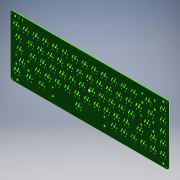
# Autodesk Inventor part: 60pc_pcb.kicad_pcb_Outline
Saved by Autodesk Inventor 2018 (Build 220112000, 112)
## iProperties
Created: 2018-02-05
Part Number: 60pc_pcb.kicad_pcb_Outline
Material: Generic
Document SubType Name: Modeling
Designer: ConnorDevitt
Density: 1 g/cm^3
Appearance: Board Outline
Author: ConnorDevitt
Autodesk Inventor part; units mm, degrees
(part 1 of 2)
ref_plane "YZ Plane" through (0, 0, 0) normal (1, 0, 0) x (0, 1, 0)
ref_plane "XZ Plane" through (0, 0, 0) normal (0, 1, 0) x (-1, 0, 0)
ref_plane "XY Plane" through (0, 0, 0) normal (0, 0, 1) x (1, 0, 0)
sketch "Sketch1" plane through (0, 0, 0) normal (0, 0, 1) x (1, 0, 0)
  line L0 (-153.25, 55.25) -> (-153.25, -54)
  arc A0 (-153.25, -54) -> (-149.25, -58) centre (-149.25, -54) ccw
  line L1 (-149.25, -58) -> (149.25, -58)
  arc A1 (149.25, -58) -> (153.25, -54) centre (149.25, -54) ccw
  line L2 (153.25, -54) -> (153.25, -53.25)
  line L3 (153.25, -53.25) -> (153.25, 55.25)
  arc A2 (153.25, 55.25) -> (150.5, 58) centre (150.5, 55.25) ccw
  line L4 (150.5, 58) -> (-150.5, 58)
  arc A3 (-150.5, 58) -> (-153.25, 55.25) centre (-150.5, 55.25) ccw
  line L5 (-126.1877, 42.5233) -> (-126.9986, 41.0634)
  arc A4 (-128.3099, 41.7917) -> (-126.9986, 41.0634) centre (-127.6542, 41.4275) ccw
  line L6 (-128.3099, 41.7917) -> (-127.4989, 43.2516)
  arc A5 (-126.1877, 42.5233) -> (-127.4989, 43.2516) centre (-126.8433, 42.8875) ccw
  line L7 (-120.5558, 43.9158) -> (-120.5952, 43.3372)
  arc A6 (-122.0917, 43.4392) -> (-120.5952, 43.3372) centre (-121.3435, 43.3882) ccw
  line L8 (-122.0917, 43.4392) -> (-122.0523, 44.0178)
  arc A7 (-120.5558, 43.9158) -> (-122.0523, 44.0178) centre (-121.304, 43.9668) ccw
  line L9 (-136.55, 55.15) -> (-136.55, 52.65)
  arc A8 (-137.25, 52.65) -> (-136.55, 52.65) centre (-136.9, 52.65) ccw
  line L10 (-137.25, 52.65) -> (-137.25, 55.15)
  arc A9 (-136.55, 55.15) -> (-137.25, 55.15) centre (-136.9, 55.15) ccw
  line L11 (-129.25, 55.15) -> (-129.25, 52.65)
  arc A10 (-129.95, 52.65) -> (-129.25, 52.65) centre (-129.6, 52.65) ccw
  line L12 (-129.95, 52.65) -> (-129.95, 55.15)
  arc A11 (-129.25, 55.15) -> (-129.95, 55.15) centre (-129.6, 55.15) ccw
  line L13 (-145.2377, 42.5233) -> (-146.0486, 41.0634)
  arc A12 (-147.3598, 41.7917) -> (-146.0486, 41.0634) centre (-146.7042, 41.4275) ccw
  line L14 (-147.3598, 41.7917) -> (-146.5489, 43.2516)
  arc A13 (-145.2377, 42.5233) -> (-146.5489, 43.2516) centre (-145.8933, 42.8875) ccw
  line L15 (-139.6058, 43.9158) -> (-139.6452, 43.3372)
  arc A14 (-141.1417, 43.4392) -> (-139.6452, 43.3372) centre (-140.3935, 43.3882) ccw
  line L16 (-141.1417, 43.4392) -> (-141.1023, 44.0178)
  arc A15 (-139.6058, 43.9158) -> (-141.1023, 44.0178) centre (-140.354, 43.9668) ccw
  line L17 (-140.4752, 23.4733) -> (-141.2861, 22.0134)
  arc A16 (-142.5974, 22.7417) -> (-141.2861, 22.0134) centre (-141.9417, 22.3775) ccw
  line L18 (-142.5974, 22.7417) -> (-141.7864, 24.2016)
  arc A17 (-140.4752, 23.4733) -> (-141.7864, 24.2016) centre (-141.1308, 23.8375) ccw
  line L19 (-134.8433, 24.8658) -> (-134.8827, 24.2872)
  arc A18 (-136.3792, 24.3892) -> (-134.8827, 24.2872) centre (-135.631, 24.3382) ccw
  line L20 (-136.3792, 24.3892) -> (-136.3398, 24.9678)
  arc A19 (-134.8433, 24.8658) -> (-136.3398, 24.9678) centre (-135.5915, 24.9168) ccw
  line L21 (-138.0939, 4.4233) -> (-138.9048, 2.9634)
  arc A20 (-140.2161, 3.6917) -> (-138.9048, 2.9634) centre (-139.5605, 3.3275) ccw
  line L22 (-140.2161, 3.6917) -> (-139.4052, 5.1516)
  arc A21 (-138.0939, 4.4233) -> (-139.4052, 5.1516) centre (-138.7495, 4.7875) ccw
  line L23 (-132.462, 5.8158) -> (-132.5015, 5.2372)
  arc A22 (-133.998, 5.3392) -> (-132.5015, 5.2372) centre (-133.2497, 5.2882) ccw
  line L24 (-133.998, 5.3392) -> (-133.9585, 5.9178)
  arc A23 (-132.462, 5.8158) -> (-133.9585, 5.9178) centre (-133.2103, 5.8668) ccw
  line L25 (-133.3314, -14.6267) -> (-134.1423, -16.0866)
  arc A24 (-135.4536, -15.3583) -> (-134.1423, -16.0866) centre (-134.798, -15.7225) ccw
  line L26 (-135.4536, -15.3583) -> (-134.6427, -13.8984)
  arc A25 (-133.3314, -14.6267) -> (-134.6427, -13.8984) centre (-133.987, -14.2625) ccw
  line L27 (-127.6995, -13.2342) -> (-127.739, -13.8128)
  arc A26 (-129.2355, -13.7108) -> (-127.739, -13.8128) centre (-128.4872, -13.7618) ccw
  line L28 (-129.2355, -13.7108) -> (-129.196, -13.1322)
  arc A27 (-127.6995, -13.2342) -> (-129.196, -13.1322) centre (-128.4478, -13.1832) ccw
  line L29 (-142.8564, -33.6767) -> (-143.6673, -35.1366)
  arc A28 (-144.9786, -34.4083) -> (-143.6673, -35.1366) centre (-144.323, -34.7725) ccw
  line L30 (-144.9786, -34.4083) -> (-144.1677, -32.9484)
  arc A29 (-142.8564, -33.6767) -> (-144.1677, -32.9484) centre (-143.512, -33.3125) ccw
  line L31 (-137.2245, -32.2842) -> (-137.264, -32.8628)
  arc A30 (-138.7605, -32.7608) -> (-137.264, -32.8628) centre (-138.0122, -32.8118) ccw
  line L32 (-138.7605, -32.7608) -> (-138.721, -32.1822)
  arc A31 (-137.2245, -32.2842) -> (-138.721, -32.1822) centre (-137.9728, -32.2332) ccw
  line L33 (-116.6627, 23.4733) -> (-117.4736, 22.0134)
  arc A32 (-118.7849, 22.7417) -> (-117.4736, 22.0134) centre (-118.1292, 22.3775) ccw
  line L34 (-118.7849, 22.7417) -> (-117.9739, 24.2016)
  arc A33 (-116.6627, 23.4733) -> (-117.9739, 24.2016) centre (-117.3183, 23.8375) ccw
  line L35 (-111.0308, 24.8658) -> (-111.0702, 24.2872)
  arc A34 (-112.5667, 24.3892) -> (-111.0702, 24.2872) centre (-111.8185, 24.3382) ccw
  line L36 (-112.5667, 24.3892) -> (-112.5273, 24.9678)
  arc A35 (-111.0308, 24.8658) -> (-112.5273, 24.9678) centre (-111.779, 24.9168) ccw
  line L37 (-111.9002, 4.4233) -> (-112.7111, 2.9634)
  arc A36 (-114.0224, 3.6917) -> (-112.7111, 2.9634) centre (-113.3667, 3.3275) ccw
  line L38 (-114.0224, 3.6917) -> (-113.2114, 5.1516)
  arc A37 (-111.9002, 4.4233) -> (-113.2114, 5.1516) centre (-112.5558, 4.7875) ccw
  line L39 (-106.2683, 5.8158) -> (-106.3077, 5.2372)
  arc A38 (-107.8042, 5.3392) -> (-106.3077, 5.2372) centre (-107.056, 5.2882) ccw
  line L40 (-107.8042, 5.3392) -> (-107.7648, 5.9178)
  arc A39 (-106.2683, 5.8158) -> (-107.7648, 5.9178) centre (-107.0165, 5.8668) ccw
  line L41 (-102.3752, -14.6267) -> (-103.1861, -16.0866)
  arc A40 (-104.4974, -15.3583) -> (-103.1861, -16.0866) centre (-103.8417, -15.7225) ccw
  line L42 (-104.4974, -15.3583) -> (-103.6864, -13.8984)
  arc A41 (-102.3752, -14.6267) -> (-103.6864, -13.8984) centre (-103.0308, -14.2625) ccw
  line L43 (-96.7433, -13.2342) -> (-96.7827, -13.8128)
  arc A42 (-98.2792, -13.7108) -> (-96.7827, -13.8128) centre (-97.531, -13.7618) ccw
  line L44 (-98.2792, -13.7108) -> (-98.2398, -13.1322)
  arc A43 (-96.7433, -13.2342) -> (-98.2398, -13.1322) centre (-97.4915, -13.1832) ccw
  line L45 (-119.0439, -33.6767) -> (-119.8548, -35.1366)
  arc A44 (-121.1661, -34.4083) -> (-119.8548, -35.1366) centre (-120.5105, -34.7725) ccw
  line L46 (-121.1661, -34.4083) -> (-120.3552, -32.9484)
  arc A45 (-119.0439, -33.6767) -> (-120.3552, -32.9484) centre (-119.6995, -33.3125) ccw
  line L47 (-113.412, -32.2842) -> (-113.4515, -32.8628)
  arc A46 (-114.948, -32.7608) -> (-113.4515, -32.8628) centre (-114.1997, -32.8118) ccw
  line L48 (-114.948, -32.7608) -> (-114.9085, -32.1822)
  arc A47 (-113.412, -32.2842) -> (-114.9085, -32.1822) centre (-114.1603, -32.2332) ccw
  line L49 (-95.2314, -33.6767) -> (-96.0423, -35.1366)
  arc A48 (-97.3536, -34.4083) -> (-96.0423, -35.1366) centre (-96.698, -34.7725) ccw
  line L50 (-97.3536, -34.4083) -> (-96.5427, -32.9484)
  arc A49 (-95.2314, -33.6767) -> (-96.5427, -32.9484) centre (-95.887, -33.3125) ccw
  line L51 (-89.5995, -32.2842) -> (-89.639, -32.8628)
  arc A50 (-91.1355, -32.7608) -> (-89.639, -32.8628) centre (-90.3872, -32.8118) ccw
  line L52 (-91.1355, -32.7608) -> (-91.096, -32.1822)
  arc A51 (-89.5995, -32.2842) -> (-91.096, -32.1822) centre (-90.3478, -32.2332) ccw
  line L53 (-107.1377, 42.5233) -> (-107.9486, 41.0634)
  arc A52 (-109.2599, 41.7917) -> (-107.9486, 41.0634) centre (-108.6042, 41.4275) ccw
  line L54 (-109.2599, 41.7917) -> (-108.4489, 43.2516)
  arc A53 (-107.1377, 42.5233) -> (-108.4489, 43.2516) centre (-107.7933, 42.8875) ccw
  line L55 (-101.5058, 43.9158) -> (-101.5452, 43.3372)
  arc A54 (-103.0417, 43.4392) -> (-101.5452, 43.3372) centre (-102.2935, 43.3882) ccw
  line L56 (-103.0417, 43.4392) -> (-103.0023, 44.0178)
  arc A55 (-101.5058, 43.9158) -> (-103.0023, 44.0178) centre (-102.254, 43.9668) ccw
  line L57 (-97.6127, 23.4733) -> (-98.4236, 22.0134)
  arc A56 (-99.7348, 22.7417) -> (-98.4236, 22.0134) centre (-99.0792, 22.3775) ccw
  line L58 (-99.7348, 22.7417) -> (-98.9239, 24.2016)
  arc A57 (-97.6127, 23.4733) -> (-98.9239, 24.2016) centre (-98.2683, 23.8375) ccw
  line L59 (-91.9808, 24.8658) -> (-92.0202, 24.2872)
  arc A58 (-93.5167, 24.3892) -> (-92.0202, 24.2872) centre (-92.7685, 24.3382) ccw
  line L60 (-93.5167, 24.3892) -> (-93.4773, 24.9678)
  arc A59 (-91.9808, 24.8658) -> (-93.4773, 24.9678) centre (-92.729, 24.9168) ccw
  line L61 (-92.8501, 4.4233) -> (-93.6611, 2.9634)
  arc A60 (-94.9724, 3.6917) -> (-93.6611, 2.9634) centre (-94.3167, 3.3275) ccw
  line L62 (-94.9724, 3.6917) -> (-94.1614, 5.1516)
  arc A61 (-92.8501, 4.4233) -> (-94.1614, 5.1516) centre (-93.5058, 4.7875) ccw
  line L63 (-87.2183, 5.8158) -> (-87.2577, 5.2372)
  arc A62 (-88.7542, 5.3392) -> (-87.2577, 5.2372) centre (-88.006, 5.2882) ccw
  line L64 (-88.7542, 5.3392) -> (-88.7148, 5.9178)
  arc A63 (-87.2183, 5.8158) -> (-88.7148, 5.9178) centre (-87.9665, 5.8668) ccw
  line L65 (-83.3251, -14.6267) -> (-84.1361, -16.0866)
  arc A64 (-85.4474, -15.3583) -> (-84.1361, -16.0866) centre (-84.7917, -15.7225) ccw
  line L66 (-85.4474, -15.3583) -> (-84.6364, -13.8984)
  arc A65 (-83.3251, -14.6267) -> (-84.6364, -13.8984) centre (-83.9808, -14.2625) ccw
  line L67 (-77.6933, -13.2342) -> (-77.7327, -13.8128)
  arc A66 (-79.2292, -13.7108) -> (-77.7327, -13.8128) centre (-78.481, -13.7618) ccw
  line L68 (-79.2292, -13.7108) -> (-79.1898, -13.1322)
  arc A67 (-77.6933, -13.2342) -> (-79.1898, -13.1322) centre (-78.4415, -13.1832) ccw
  line L69 (-88.0876, 42.5233) -> (-88.8986, 41.0634)
  arc A68 (-90.2099, 41.7917) -> (-88.8986, 41.0634) centre (-89.5542, 41.4275) ccw
  line L70 (-90.2099, 41.7917) -> (-89.3989, 43.2516)
  arc A69 (-88.0876, 42.5233) -> (-89.3989, 43.2516) centre (-88.7433, 42.8875) ccw
  line L71 (-82.4558, 43.9158) -> (-82.4952, 43.3372)
  arc A70 (-83.9917, 43.4392) -> (-82.4952, 43.3372) centre (-83.2435, 43.3882) ccw
  line L72 (-83.9917, 43.4392) -> (-83.9523, 44.0178)
  arc A71 (-82.4558, 43.9158) -> (-83.9523, 44.0178) centre (-83.204, 43.9668) ccw
  line L73 (-78.5627, 23.4733) -> (-79.3736, 22.0134)
  arc A72 (-80.6849, 22.7417) -> (-79.3736, 22.0134) centre (-80.0292, 22.3775) ccw
  line L74 (-80.6849, 22.7417) -> (-79.8739, 24.2016)
  arc A73 (-78.5627, 23.4733) -> (-79.8739, 24.2016) centre (-79.2183, 23.8375) ccw
  line L75 (-72.9308, 24.8658) -> (-72.9702, 24.2872)
  arc A74 (-74.4667, 24.3892) -> (-72.9702, 24.2872) centre (-73.7185, 24.3382) ccw
  line L76 (-74.4667, 24.3892) -> (-74.4273, 24.9678)
  arc A75 (-72.9308, 24.8658) -> (-74.4273, 24.9678) centre (-73.679, 24.9168) ccw
  line L77 (-73.8002, 4.4233) -> (-74.6111, 2.9634)
  arc A76 (-75.9223, 3.6917) -> (-74.6111, 2.9634) centre (-75.2667, 3.3275) ccw
  line L78 (-75.9223, 3.6917) -> (-75.1114, 5.1516)
  arc A77 (-73.8002, 4.4233) -> (-75.1114, 5.1516) centre (-74.4558, 4.7875) ccw
  line L79 (-68.1683, 5.8158) -> (-68.2077, 5.2372)
  arc A78 (-69.7042, 5.3392) -> (-68.2077, 5.2372) centre (-68.956, 5.2882) ccw
  line L80 (-69.7042, 5.3392) -> (-69.6648, 5.9178)
  arc A79 (-68.1683, 5.8158) -> (-69.6648, 5.9178) centre (-68.9165, 5.8668) ccw
  line L81 (-64.2751, -14.6267) -> (-65.0861, -16.0866)
  arc A80 (-66.3974, -15.3583) -> (-65.0861, -16.0866) centre (-65.7417, -15.7225) ccw
  line L82 (-66.3974, -15.3583) -> (-65.5864, -13.8984)
  arc A81 (-64.2751, -14.6267) -> (-65.5864, -13.8984) centre (-64.9308, -14.2625) ccw
  line L83 (-58.6433, -13.2342) -> (-58.6827, -13.8128)
  arc A82 (-60.1792, -13.7108) -> (-58.6827, -13.8128) centre (-59.431, -13.7618) ccw
  line L84 (-60.1792, -13.7108) -> (-60.1398, -13.1322)
  arc A83 (-58.6433, -13.2342) -> (-60.1398, -13.1322) centre (-59.3915, -13.1832) ccw
  line L85 (-69.0376, 42.5233) -> (-69.8486, 41.0634)
  arc A84 (-71.1599, 41.7917) -> (-69.8486, 41.0634) centre (-70.5042, 41.4275) ccw
  line L86 (-71.1599, 41.7917) -> (-70.3489, 43.2516)
  arc A85 (-69.0376, 42.5233) -> (-70.3489, 43.2516) centre (-69.6933, 42.8875) ccw
  line L87 (-63.4058, 43.9158) -> (-63.4452, 43.3372)
  arc A86 (-64.9417, 43.4392) -> (-63.4452, 43.3372) centre (-64.1935, 43.3882) ccw
  line L88 (-64.9417, 43.4392) -> (-64.9023, 44.0178)
  arc A87 (-63.4058, 43.9158) -> (-64.9023, 44.0178) centre (-64.154, 43.9668) ccw
  line L89 (-59.5127, 23.4733) -> (-60.3236, 22.0134)
  arc A88 (-61.6349, 22.7417) -> (-60.3236, 22.0134) centre (-60.9792, 22.3775) ccw
  line L90 (-61.6349, 22.7417) -> (-60.8239, 24.2016)
  arc A89 (-59.5127, 23.4733) -> (-60.8239, 24.2016) centre (-60.1683, 23.8375) ccw
  line L91 (-53.8808, 24.8658) -> (-53.9202, 24.2872)
  arc A90 (-55.4167, 24.3892) -> (-53.9202, 24.2872) centre (-54.6685, 24.3382) ccw
  line L92 (-55.4167, 24.3892) -> (-55.3773, 24.9678)
  arc A91 (-53.8808, 24.8658) -> (-55.3773, 24.9678) centre (-54.629, 24.9168) ccw
  line L93 (-54.7501, 4.4233) -> (-55.5611, 2.9634)
  arc A92 (-56.8724, 3.6917) -> (-55.5611, 2.9634) centre (-56.2167, 3.3275) ccw
  line L94 (-56.8724, 3.6917) -> (-56.0614, 5.1516)
  arc A93 (-54.7501, 4.4233) -> (-56.0614, 5.1516) centre (-55.4058, 4.7875) ccw
  line L95 (-49.1183, 5.8158) -> (-49.1577, 5.2372)
  arc A94 (-50.6542, 5.3392) -> (-49.1577, 5.2372) centre (-49.906, 5.2882) ccw
  line L96 (-50.6542, 5.3392) -> (-50.6148, 5.9178)
  arc A95 (-49.1183, 5.8158) -> (-50.6148, 5.9178) centre (-49.8665, 5.8668) ccw
  line L97 (-45.2251, -14.6267) -> (-46.0361, -16.0866)
  arc A96 (-47.3473, -15.3583) -> (-46.0361, -16.0866) centre (-46.6917, -15.7225) ccw
  line L98 (-47.3473, -15.3583) -> (-46.5364, -13.8984)
  arc A97 (-45.2251, -14.6267) -> (-46.5364, -13.8984) centre (-45.8808, -14.2625) ccw
  line L99 (-39.5933, -13.2342) -> (-39.6327, -13.8128)
  arc A98 (-41.1292, -13.7108) -> (-39.6327, -13.8128) centre (-40.381, -13.7618) ccw
  line L100 (-41.1292, -13.7108) -> (-41.0898, -13.1322)
  arc A99 (-39.5933, -13.2342) -> (-41.0898, -13.1322) centre (-40.3415, -13.1832) ccw
  line L101 (-49.9877, 42.5233) -> (-50.7986, 41.0634)
  arc A100 (-52.1099, 41.7917) -> (-50.7986, 41.0634) centre (-51.4542, 41.4275) ccw
  line L102 (-52.1099, 41.7917) -> (-51.2989, 43.2516)
  arc A101 (-49.9877, 42.5233) -> (-51.2989, 43.2516) centre (-50.6433, 42.8875) ccw
  line L103 (-44.3558, 43.9158) -> (-44.3952, 43.3372)
  arc A102 (-45.8917, 43.4392) -> (-44.3952, 43.3372) centre (-45.1435, 43.3882) ccw
  line L104 (-45.8917, 43.4392) -> (-45.8523, 44.0178)
  arc A103 (-44.3558, 43.9158) -> (-45.8523, 44.0178) centre (-45.104, 43.9668) ccw
  line L105 (-40.4626, 23.4733) -> (-41.2736, 22.0134)
  arc A104 (-42.5849, 22.7417) -> (-41.2736, 22.0134) centre (-41.9292, 22.3775) ccw
  line L106 (-42.5849, 22.7417) -> (-41.7739, 24.2016)
  arc A105 (-40.4626, 23.4733) -> (-41.7739, 24.2016) centre (-41.1183, 23.8375) ccw
  line L107 (-34.8308, 24.8658) -> (-34.8702, 24.2872)
  arc A106 (-36.3667, 24.3892) -> (-34.8702, 24.2872) centre (-35.6185, 24.3382) ccw
  line L108 (-36.3667, 24.3892) -> (-36.3273, 24.9678)
  arc A107 (-34.8308, 24.8658) -> (-36.3273, 24.9678) centre (-35.579, 24.9168) ccw
  line L109 (-35.7002, 4.4233) -> (-36.5111, 2.9634)
  arc A108 (-37.8224, 3.6917) -> (-36.5111, 2.9634) centre (-37.1667, 3.3275) ccw
  line L110 (-37.8224, 3.6917) -> (-37.0114, 5.1516)
  arc A109 (-35.7002, 4.4233) -> (-37.0114, 5.1516) centre (-36.3558, 4.7875) ccw
  line L111 (-30.0683, 5.8158) -> (-30.1077, 5.2372)
  arc A110 (-31.6042, 5.3392) -> (-30.1077, 5.2372) centre (-30.856, 5.2882) ccw
  line L112 (-31.6042, 5.3392) -> (-31.5648, 5.9178)
  arc A111 (-30.0683, 5.8158) -> (-31.5648, 5.9178) centre (-30.8165, 5.8668) ccw
  line L113 (-26.1752, -14.6267) -> (-26.9861, -16.0866)
  arc A112 (-28.2974, -15.3583) -> (-26.9861, -16.0866) centre (-27.6417, -15.7225) ccw
  line L114 (-28.2974, -15.3583) -> (-27.4864, -13.8984)
  arc A113 (-26.1752, -14.6267) -> (-27.4864, -13.8984) centre (-26.8308, -14.2625) ccw
  line L115 (-20.5433, -13.2342) -> (-20.5827, -13.8128)
  arc A114 (-22.0792, -13.7108) -> (-20.5827, -13.8128) centre (-21.331, -13.7618) ccw
  line L116 (-22.0792, -13.7108) -> (-22.0398, -13.1322)
  arc A115 (-20.5433, -13.2342) -> (-22.0398, -13.1322) centre (-21.2915, -13.1832) ccw
  line L117 (-30.9377, 42.5233) -> (-31.7486, 41.0634)
  arc A116 (-33.0598, 41.7917) -> (-31.7486, 41.0634) centre (-32.4042, 41.4275) ccw
  line L118 (-33.0598, 41.7917) -> (-32.2489, 43.2516)
  arc A117 (-30.9377, 42.5233) -> (-32.2489, 43.2516) centre (-31.5933, 42.8875) ccw
  line L119 (-25.3058, 43.9158) -> (-25.3452, 43.3372)
  arc A118 (-26.8417, 43.4392) -> (-25.3452, 43.3372) centre (-26.0935, 43.3882) ccw
  line L120 (-26.8417, 43.4392) -> (-26.8023, 44.0178)
  arc A119 (-25.3058, 43.9158) -> (-26.8023, 44.0178) centre (-26.054, 43.9668) ccw
  line L121 (-21.4127, 23.4733) -> (-22.2236, 22.0134)
  arc A120 (-23.5348, 22.7417) -> (-22.2236, 22.0134) centre (-22.8792, 22.3775) ccw
  line L122 (-23.5348, 22.7417) -> (-22.7239, 24.2016)
  arc A121 (-21.4127, 23.4733) -> (-22.7239, 24.2016) centre (-22.0683, 23.8375) ccw
  line L123 (-15.7808, 24.8658) -> (-15.8202, 24.2872)
  arc A122 (-17.3167, 24.3892) -> (-15.8202, 24.2872) centre (-16.5685, 24.3382) ccw
  line L124 (-17.3167, 24.3892) -> (-17.2773, 24.9678)
  arc A123 (-15.7808, 24.8658) -> (-17.2773, 24.9678) centre (-16.529, 24.9168) ccw
  line L125 (-16.6502, 4.4233) -> (-17.4611, 2.9634)
  arc A124 (-18.7723, 3.6917) -> (-17.4611, 2.9634) centre (-18.1167, 3.3275) ccw
  line L126 (-18.7723, 3.6917) -> (-17.9614, 5.1516)
  arc A125 (-16.6502, 4.4233) -> (-17.9614, 5.1516) centre (-17.3058, 4.7875) ccw
  line L127 (-11.0183, 5.8158) -> (-11.0577, 5.2372)
  arc A126 (-12.5542, 5.3392) -> (-11.0577, 5.2372) centre (-11.806, 5.2882) ccw
  line L128 (-12.5542, 5.3392) -> (-12.5148, 5.9178)
  arc A127 (-11.0183, 5.8158) -> (-12.5148, 5.9178) centre (-11.7665, 5.8668) ccw
  line L129 (-7.1251, -14.6267) -> (-7.9361, -16.0866)
  arc A128 (-9.2474, -15.3583) -> (-7.9361, -16.0866) centre (-8.5917, -15.7225) ccw
  line L130 (-9.2474, -15.3583) -> (-8.4364, -13.8984)
  arc A129 (-7.1251, -14.6267) -> (-8.4364, -13.8984) centre (-7.7808, -14.2625) ccw
  line L131 (-1.4933, -13.2342) -> (-1.5327, -13.8128)
  arc A130 (-3.0292, -13.7108) -> (-1.5327, -13.8128) centre (-2.281, -13.7618) ccw
  line L132 (-3.0292, -13.7108) -> (-2.9898, -13.1322)
  arc A131 (-1.4933, -13.2342) -> (-2.9898, -13.1322) centre (-2.2415, -13.1832) ccw
  line L133 (-23.7939, -33.6767) -> (-24.6048, -35.1366)
  arc A132 (-25.9161, -34.4083) -> (-24.6048, -35.1366) centre (-25.2605, -34.7725) ccw
  line L134 (-25.9161, -34.4083) -> (-25.1052, -32.9484)
  arc A133 (-23.7939, -33.6767) -> (-25.1052, -32.9484) centre (-24.4495, -33.3125) ccw
  line L135 (-18.162, -32.2842) -> (-18.2015, -32.8628)
  arc A134 (-19.698, -32.7608) -> (-18.2015, -32.8628) centre (-18.9497, -32.8118) ccw
  line L136 (-19.698, -32.7608) -> (-19.6585, -32.1822)
  arc A135 (-18.162, -32.2842) -> (-19.6585, -32.1822) centre (-18.9103, -32.2332) ccw
  line L137 (-11.8877, 42.5233) -> (-12.6986, 41.0634)
  arc A136 (-14.0099, 41.7917) -> (-12.6986, 41.0634) centre (-13.3542, 41.4275) ccw
  line L138 (-14.0099, 41.7917) -> (-13.1989, 43.2516)
  arc A137 (-11.8877, 42.5233) -> (-13.1989, 43.2516) centre (-12.5433, 42.8875) ccw
  line L139 (-6.2558, 43.9158) -> (-6.2952, 43.3372)
  arc A138 (-7.7917, 43.4392) -> (-6.2952, 43.3372) centre (-7.0435, 43.3882) ccw
  line L140 (-7.7917, 43.4392) -> (-7.7523, 44.0178)
  arc A139 (-6.2558, 43.9158) -> (-7.7523, 44.0178) centre (-7.004, 43.9668) ccw
  line L141 (-2.3626, 23.4733) -> (-3.1736, 22.0134)
  arc A140 (-4.4848, 22.7417) -> (-3.1736, 22.0134) centre (-3.8292, 22.3775) ccw
  line L142 (-4.4848, 22.7417) -> (-3.6739, 24.2016)
  arc A141 (-2.3626, 23.4733) -> (-3.6739, 24.2016) centre (-3.0183, 23.8375) ccw
  line L143 (3.2692, 24.8658) -> (3.2298, 24.2872)
  arc A142 (1.7333, 24.3892) -> (3.2298, 24.2872) centre (2.4815, 24.3382) ccw
  line L144 (1.7333, 24.3892) -> (1.7727, 24.9678)
  arc A143 (3.2692, 24.8658) -> (1.7727, 24.9678) centre (2.521, 24.9168) ccw
  line L145 (2.3998, 4.4233) -> (1.5889, 2.9634)
  arc A144 (0.2777, 3.6917) -> (1.5889, 2.9634) centre (0.9333, 3.3275) ccw
  line L146 (0.2777, 3.6917) -> (1.0886, 5.1516)
  arc A145 (2.3998, 4.4233) -> (1.0886, 5.1516) centre (1.7442, 4.7875) ccw
  line L147 (8.0317, 5.8158) -> (7.9923, 5.2372)
  arc A146 (6.4958, 5.3392) -> (7.9923, 5.2372) centre (7.244, 5.2882) ccw
  line L148 (6.4958, 5.3392) -> (6.5352, 5.9178)
  arc A147 (8.0317, 5.8158) -> (6.5352, 5.9178) centre (7.2835, 5.8668) ccw
  line L149 (11.9248, -14.6267) -> (11.1139, -16.0866)
  arc A148 (9.8026, -15.3583) -> (11.1139, -16.0866) centre (10.4583, -15.7225) ccw
  line L150 (9.8026, -15.3583) -> (10.6136, -13.8984)
  arc A149 (11.9248, -14.6267) -> (10.6136, -13.8984) centre (11.2692, -14.2625) ccw
  line L151 (17.5567, -13.2342) -> (17.5173, -13.8128)
  arc A150 (16.0208, -13.7108) -> (17.5173, -13.8128) centre (16.769, -13.7618) ccw
  line L152 (16.0208, -13.7108) -> (16.0602, -13.1322)
  arc A151 (17.5567, -13.2342) -> (16.0602, -13.1322) centre (16.8085, -13.1832) ccw
  line L153 (7.1624, 42.5233) -> (6.3514, 41.0634)
  arc A152 (5.0401, 41.7917) -> (6.3514, 41.0634) centre (5.6958, 41.4275) ccw
  line L154 (5.0401, 41.7917) -> (5.8511, 43.2516)
  arc A153 (7.1624, 42.5233) -> (5.8511, 43.2516) centre (6.5067, 42.8875) ccw
  line L155 (12.7942, 43.9158) -> (12.7548, 43.3372)
  arc A154 (11.2583, 43.4392) -> (12.7548, 43.3372) centre (12.0065, 43.3882) ccw
  line L156 (11.2583, 43.4392) -> (11.2977, 44.0178)
  arc A155 (12.7942, 43.9158) -> (11.2977, 44.0178) centre (12.046, 43.9668) ccw
  line L157 (16.6873, 23.4733) -> (15.8764, 22.0134)
  arc A156 (14.5651, 22.7417) -> (15.8764, 22.0134) centre (15.2208, 22.3775) ccw
  line L158 (14.5651, 22.7417) -> (15.3761, 24.2016)
  arc A157 (16.6873, 23.4733) -> (15.3761, 24.2016) centre (16.0317, 23.8375) ccw
  line L159 (22.3192, 24.8658) -> (22.2798, 24.2872)
  arc A158 (20.7833, 24.3892) -> (22.2798, 24.2872) centre (21.5315, 24.3382) ccw
  line L160 (20.7833, 24.3892) -> (20.8227, 24.9678)
  arc A159 (22.3192, 24.8658) -> (20.8227, 24.9678) centre (21.571, 24.9168) ccw
  line L161 (21.4499, 4.4233) -> (20.6389, 2.9634)
  arc A160 (19.3276, 3.6917) -> (20.6389, 2.9634) centre (19.9833, 3.3275) ccw
  line L162 (19.3276, 3.6917) -> (20.1386, 5.1516)
  arc A161 (21.4499, 4.4233) -> (20.1386, 5.1516) centre (20.7942, 4.7875) ccw
  line L163 (27.0817, 5.8158) -> (27.0423, 5.2372)
  arc A162 (25.5458, 5.3392) -> (27.0423, 5.2372) centre (26.294, 5.2882) ccw
  line L164 (25.5458, 5.3392) -> (25.5852, 5.9178)
  arc A163 (27.0817, 5.8158) -> (25.5852, 5.9178) centre (26.3335, 5.8668) ccw
  line L165 (30.9749, -14.6267) -> (30.1639, -16.0866)
  arc A164 (28.8527, -15.3583) -> (30.1639, -16.0866) centre (29.5083, -15.7225) ccw
  line L166 (28.8527, -15.3583) -> (29.6636, -13.8984)
  arc A165 (30.9749, -14.6267) -> (29.6636, -13.8984) centre (30.3192, -14.2625) ccw
  line L167 (36.6067, -13.2342) -> (36.5673, -13.8128)
  arc A166 (35.0708, -13.7108) -> (36.5673, -13.8128) centre (35.819, -13.7618) ccw
  line L168 (35.0708, -13.7108) -> (35.1102, -13.1322)
  arc A167 (36.6067, -13.2342) -> (35.1102, -13.1322) centre (35.8585, -13.1832) ccw
  line L169 (26.2124, 42.5233) -> (25.4014, 41.0634)
  arc A168 (24.0902, 41.7917) -> (25.4014, 41.0634) centre (24.7458, 41.4275) ccw
  line L170 (24.0902, 41.7917) -> (24.9011, 43.2516)
  arc A169 (26.2124, 42.5233) -> (24.9011, 43.2516) centre (25.5567, 42.8875) ccw
  line L171 (31.8442, 43.9158) -> (31.8048, 43.3372)
  arc A170 (30.3083, 43.4392) -> (31.8048, 43.3372) centre (31.0565, 43.3882) ccw
  line L172 (30.3083, 43.4392) -> (30.3477, 44.0178)
  arc A171 (31.8442, 43.9158) -> (30.3477, 44.0178) centre (31.096, 43.9668) ccw
  line L173 (35.7373, 23.4733) -> (34.9264, 22.0134)
  arc A172 (33.6151, 22.7417) -> (34.9264, 22.0134) centre (34.2708, 22.3775) ccw
  line L174 (33.6151, 22.7417) -> (34.4261, 24.2016)
  arc A173 (35.7373, 23.4733) -> (34.4261, 24.2016) centre (35.0817, 23.8375) ccw
  line L175 (41.3692, 24.8658) -> (41.3298, 24.2872)
  arc A174 (39.8333, 24.3892) -> (41.3298, 24.2872) centre (40.5815, 24.3382) ccw
  line L176 (39.8333, 24.3892) -> (39.8727, 24.9678)
  arc A175 (41.3692, 24.8658) -> (39.8727, 24.9678) centre (40.621, 24.9168) ccw
  line L177 (40.4999, 4.4233) -> (39.6889, 2.9634)
  arc A176 (38.3777, 3.6917) -> (39.6889, 2.9634) centre (39.0333, 3.3275) ccw
  line L178 (38.3777, 3.6917) -> (39.1886, 5.1516)
  arc A177 (40.4999, 4.4233) -> (39.1886, 5.1516) centre (39.8442, 4.7875) ccw
  line L179 (46.1317, 5.8158) -> (46.0923, 5.2372)
  arc A178 (44.5958, 5.3392) -> (46.0923, 5.2372) centre (45.344, 5.2882) ccw
  line L180 (44.5958, 5.3392) -> (44.6352, 5.9178)
  arc A179 (46.1317, 5.8158) -> (44.6352, 5.9178) centre (45.3835, 5.8668) ccw
  line L181 (50.0249, -14.6267) -> (49.2139, -16.0866)
  arc A180 (47.9027, -15.3583) -> (49.2139, -16.0866) centre (48.5583, -15.7225) ccw
  line L182 (47.9027, -15.3583) -> (48.7136, -13.8984)
  arc A181 (50.0249, -14.6267) -> (48.7136, -13.8984) centre (49.3692, -14.2625) ccw
  line L183 (55.6567, -13.2342) -> (55.6173, -13.8128)
  arc A182 (54.1208, -13.7108) -> (55.6173, -13.8128) centre (54.869, -13.7618) ccw
  line L184 (54.1208, -13.7108) -> (54.1602, -13.1322)
  arc A183 (55.6567, -13.2342) -> (54.1602, -13.1322) centre (54.9085, -13.1832) ccw
  line L185 (45.2623, 42.5233) -> (44.4514, 41.0634)
  arc A184 (43.1402, 41.7917) -> (44.4514, 41.0634) centre (43.7958, 41.4275) ccw
  line L186 (43.1402, 41.7917) -> (43.9511, 43.2516)
  arc A185 (45.2623, 42.5233) -> (43.9511, 43.2516) centre (44.6067, 42.8875) ccw
  line L187 (50.8942, 43.9158) -> (50.8548, 43.3372)
  arc A186 (49.3583, 43.4392) -> (50.8548, 43.3372) centre (50.1065, 43.3882) ccw
  line L188 (49.3583, 43.4392) -> (49.3977, 44.0178)
  arc A187 (50.8942, 43.9158) -> (49.3977, 44.0178) centre (50.146, 43.9668) ccw
  line L189 (54.7874, 23.4733) -> (53.9764, 22.0134)
  arc A188 (52.6651, 22.7417) -> (53.9764, 22.0134) centre (53.3208, 22.3775) ccw
  line L190 (52.6651, 22.7417) -> (53.4761, 24.2016)
  arc A189 (54.7874, 23.4733) -> (53.4761, 24.2016) centre (54.1317, 23.8375) ccw
  line L191 (60.4192, 24.8658) -> (60.3798, 24.2872)
  arc A190 (58.8833, 24.3892) -> (60.3798, 24.2872) centre (59.6315, 24.3382) ccw
  line L192 (58.8833, 24.3892) -> (58.9227, 24.9678)
  arc A191 (60.4192, 24.8658) -> (58.9227, 24.9678) centre (59.671, 24.9168) ccw
  line L193 (59.5499, 4.4233) -> (58.7389, 2.9634)
  arc A192 (57.4276, 3.6917) -> (58.7389, 2.9634) centre (58.0833, 3.3275) ccw
  line L194 (57.4276, 3.6917) -> (58.2386, 5.1516)
  arc A193 (59.5499, 4.4233) -> (58.2386, 5.1516) centre (58.8942, 4.7875) ccw
  line L195 (65.1817, 5.8158) -> (65.1423, 5.2372)
  arc A194 (63.6458, 5.3392) -> (65.1423, 5.2372) centre (64.394, 5.2882) ccw
  line L196 (63.6458, 5.3392) -> (63.6852, 5.9178)
  arc A195 (65.1817, 5.8158) -> (63.6852, 5.9178) centre (64.4335, 5.8668) ccw
  line L197 (69.0748, -14.6267) -> (68.2639, -16.0866)
  arc A196 (66.9527, -15.3583) -> (68.2639, -16.0866) centre (67.6083, -15.7225) ccw
  line L198 (66.9527, -15.3583) -> (67.7636, -13.8984)
  arc A197 (69.0748, -14.6267) -> (67.7636, -13.8984) centre (68.4192, -14.2625) ccw
  line L199 (74.7067, -13.2342) -> (74.6673, -13.8128)
  arc A198 (73.1708, -13.7108) -> (74.6673, -13.8128) centre (73.919, -13.7618) ccw
  line L200 (73.1708, -13.7108) -> (73.2102, -13.1322)
  arc A199 (74.7067, -13.2342) -> (73.2102, -13.1322) centre (73.9585, -13.1832) ccw
  line L201 (45.2623, -33.6767) -> (44.4514, -35.1366)
  arc A200 (43.1402, -34.4083) -> (44.4514, -35.1366) centre (43.7958, -34.7725) ccw
  line L202 (43.1402, -34.4083) -> (43.9511, -32.9484)
  arc A201 (45.2623, -33.6767) -> (43.9511, -32.9484) centre (44.6067, -33.3125) ccw
  line L203 (50.8942, -32.2842) -> (50.8548, -32.8628)
  arc A202 (49.3583, -32.7608) -> (50.8548, -32.8628) centre (50.1065, -32.8118) ccw
  line L204 (49.3583, -32.7608) -> (49.3977, -32.1822)
  arc A203 (50.8942, -32.2842) -> (49.3977, -32.1822) centre (50.146, -32.2332) ccw
  line L205 (64.3123, 42.5233) -> (63.5014, 41.0634)
  arc A204 (62.1902, 41.7917) -> (63.5014, 41.0634) centre (62.8458, 41.4275) ccw
  line L206 (62.1902, 41.7917) -> (63.0011, 43.2516)
  arc A205 (64.3123, 42.5233) -> (63.0011, 43.2516) centre (63.6567, 42.8875) ccw
  line L207 (69.9442, 43.9158) -> (69.9048, 43.3372)
  arc A206 (68.4083, 43.4392) -> (69.9048, 43.3372) centre (69.1565, 43.3882) ccw
  line L208 (68.4083, 43.4392) -> (68.4477, 44.0178)
  arc A207 (69.9442, 43.9158) -> (68.4477, 44.0178) centre (69.196, 43.9668) ccw
  line L209 (73.8374, 23.4733) -> (73.0264, 22.0134)
  arc A208 (71.7151, 22.7417) -> (73.0264, 22.0134) centre (72.3708, 22.3775) ccw
  line L210 (71.7151, 22.7417) -> (72.5261, 24.2016)
  arc A209 (73.8374, 23.4733) -> (72.5261, 24.2016) centre (73.1817, 23.8375) ccw
  line L211 (79.4692, 24.8658) -> (79.4298, 24.2872)
  arc A210 (77.9333, 24.3892) -> (79.4298, 24.2872) centre (78.6815, 24.3382) ccw
  line L212 (77.9333, 24.3892) -> (77.9727, 24.9678)
  arc A211 (79.4692, 24.8658) -> (77.9727, 24.9678) centre (78.721, 24.9168) ccw
  line L213 (78.5999, 4.4233) -> (77.7889, 2.9634)
  arc A212 (76.4776, 3.6917) -> (77.7889, 2.9634) centre (77.1333, 3.3275) ccw
  line L214 (76.4776, 3.6917) -> (77.2886, 5.1516)
  arc A213 (78.5999, 4.4233) -> (77.2886, 5.1516) centre (77.9442, 4.7875) ccw
  line L215 (84.2317, 5.8158) -> (84.1923, 5.2372)
  arc A214 (82.6958, 5.3392) -> (84.1923, 5.2372) centre (83.444, 5.2882) ccw
  line L216 (82.6958, 5.3392) -> (82.7352, 5.9178)
  arc A215 (84.2317, 5.8158) -> (82.7352, 5.9178) centre (83.4835, 5.8668) ccw
  line L217 (64.3123, -33.6767) -> (63.5014, -35.1366)
  arc A216 (62.1902, -34.4083) -> (63.5014, -35.1366) centre (62.8458, -34.7725) ccw
  line L218 (62.1902, -34.4083) -> (63.0011, -32.9484)
  arc A217 (64.3123, -33.6767) -> (63.0011, -32.9484) centre (63.6567, -33.3125) ccw
  line L219 (69.9442, -32.2842) -> (69.9048, -32.8628)
  arc A218 (68.4083, -32.7608) -> (69.9048, -32.8628) centre (69.1565, -32.8118) ccw
  line L220 (68.4083, -32.7608) -> (68.4477, -32.1822)
  arc A219 (69.9442, -32.2842) -> (68.4477, -32.1822) centre (69.196, -32.2332) ccw
  line L221 (83.3624, 42.5233) -> (82.5514, 41.0634)
  arc A220 (81.2401, 41.7917) -> (82.5514, 41.0634) centre (81.8958, 41.4275) ccw
  line L222 (81.2401, 41.7917) -> (82.0511, 43.2516)
  arc A221 (83.3624, 42.5233) -> (82.0511, 43.2516) centre (82.7067, 42.8875) ccw
  line L223 (88.9942, 43.9158) -> (88.9548, 43.3372)
  arc A222 (87.4583, 43.4392) -> (88.9548, 43.3372) centre (88.2065, 43.3882) ccw
  line L224 (87.4583, 43.4392) -> (87.4977, 44.0178)
  arc A223 (88.9942, 43.9158) -> (87.4977, 44.0178) centre (88.246, 43.9668) ccw
  line L225 (92.8874, 23.4733) -> (92.0764, 22.0134)
  arc A224 (90.7652, 22.7417) -> (92.0764, 22.0134) centre (91.4208, 22.3775) ccw
  line L226 (90.7652, 22.7417) -> (91.5761, 24.2016)
  arc A225 (92.8874, 23.4733) -> (91.5761, 24.2016) centre (92.2317, 23.8375) ccw
  line L227 (98.5192, 24.8658) -> (98.4798, 24.2872)
  arc A226 (96.9833, 24.3892) -> (98.4798, 24.2872) centre (97.7315, 24.3382) ccw
  line L228 (96.9833, 24.3892) -> (97.0227, 24.9678)
  arc A227 (98.5192, 24.8658) -> (97.0227, 24.9678) centre (97.771, 24.9168) ccw
  line L229 (109.5561, 4.4233) -> (108.7452, 2.9634)
  arc A228 (107.4339, 3.6917) -> (108.7452, 2.9634) centre (108.0895, 3.3275) ccw
  line L230 (107.4339, 3.6917) -> (108.2448, 5.1516)
  arc A229 (109.5561, 4.4233) -> (108.2448, 5.1516) centre (108.9005, 4.7875) ccw
  line L231 (115.188, 5.8158) -> (115.1485, 5.2372)
  arc A230 (113.652, 5.3392) -> (115.1485, 5.2372) centre (114.4003, 5.2882) ccw
  line L232 (113.652, 5.3392) -> (113.6915, 5.9178)
  arc A231 (115.188, 5.8158) -> (113.6915, 5.9178) centre (114.4397, 5.8668) ccw
  line L233 (121.4624, -14.6267) -> (120.6514, -16.0866)
  arc A232 (119.3402, -15.3583) -> (120.6514, -16.0866) centre (119.9958, -15.7225) ccw
  line L234 (119.3402, -15.3583) -> (120.1511, -13.8984)
  arc A233 (121.4624, -14.6267) -> (120.1511, -13.8984) centre (120.8067, -14.2625) ccw
  line L235 (127.0942, -13.2342) -> (127.0548, -13.8128)
  arc A234 (125.5583, -13.7108) -> (127.0548, -13.8128) centre (126.3065, -13.7618) ccw
  line L236 (125.5583, -13.7108) -> (125.5977, -13.1322)
  arc A235 (127.0942, -13.2342) -> (125.5977, -13.1322) centre (126.346, -13.1832) ccw
  line L237 (83.3624, -33.6767) -> (82.5514, -35.1366)
  arc A236 (81.2401, -34.4083) -> (82.5514, -35.1366) centre (81.8958, -34.7725) ccw
  line L238 (81.2401, -34.4083) -> (82.0511, -32.9484)
  arc A237 (83.3624, -33.6767) -> (82.0511, -32.9484) centre (82.7067, -33.3125) ccw
  line L239 (88.9942, -32.2842) -> (88.9548, -32.8628)
  arc A238 (87.4583, -32.7608) -> (88.9548, -32.8628) centre (88.2065, -32.8118) ccw
  line L240 (87.4583, -32.7608) -> (87.4977, -32.1822)
  arc A239 (88.9942, -32.2842) -> (87.4977, -32.1822) centre (88.246, -32.2332) ccw
  line L241 (111.9374, 42.5233) -> (111.1264, 41.0634)
  arc A240 (109.8152, 41.7917) -> (111.1264, 41.0634) centre (110.4708, 41.4275) ccw
  line L242 (109.8152, 41.7917) -> (110.6261, 43.2516)
  arc A241 (111.9374, 42.5233) -> (110.6261, 43.2516) centre (111.2817, 42.8875) ccw
  line L243 (117.5692, 43.9158) -> (117.5298, 43.3372)
  arc A242 (116.0333, 43.4392) -> (117.5298, 43.3372) centre (116.7815, 43.3882) ccw
  line L244 (116.0333, 43.4392) -> (116.0727, 44.0178)
  arc A243 (117.5692, 43.9158) -> (116.0727, 44.0178) centre (116.821, 43.9668) ccw
  line L245 (116.6998, 23.4733) -> (115.8889, 22.0134)
  arc A244 (114.5777, 22.7417) -> (115.8889, 22.0134) centre (115.2333, 22.3775) ccw
  line L246 (114.5777, 22.7417) -> (115.3886, 24.2016)
  arc A245 (116.6998, 23.4733) -> (115.3886, 24.2016) centre (116.0442, 23.8375) ccw
  line L247 (122.3317, 24.8658) -> (122.2923, 24.2872)
  arc A246 (120.7958, 24.3892) -> (122.2923, 24.2872) centre (121.544, 24.3382) ccw
  line L248 (120.7958, 24.3892) -> (120.8352, 24.9678)
  arc A247 (122.3317, 24.8658) -> (120.8352, 24.9678) centre (121.5835, 24.9168) ccw
  line L249 (140.5123, 4.4233) -> (139.7014, 2.9634)
  arc A248 (138.3902, 3.6917) -> (139.7014, 2.9634) centre (139.0458, 3.3275) ccw
  line L250 (138.3902, 3.6917) -> (139.2011, 5.1516)
  arc A249 (140.5123, 4.4233) -> (139.2011, 5.1516) centre (139.8567, 4.7875) ccw
  line L251 (146.1442, 5.8158) -> (146.1048, 5.2372)
  arc A250 (144.6083, 5.3392) -> (146.1048, 5.2372) centre (145.3565, 5.2882) ccw
  line L252 (144.6083, 5.3392) -> (144.6477, 5.9178)
  arc A251 (146.1442, 5.8158) -> (144.6477, 5.9178) centre (145.396, 5.8668) ccw
  line L253 (140.5123, -14.6267) -> (139.7014, -16.0866)
  arc A252 (138.3902, -15.3583) -> (139.7014, -16.0866) centre (139.0458, -15.7225) ccw
  line L254 (138.3902, -15.3583) -> (139.2011, -13.8984)
  arc A253 (140.5123, -14.6267) -> (139.2011, -13.8984) centre (139.8567, -14.2625) ccw
  line L255 (146.1442, -13.2342) -> (146.1048, -13.8128)
  arc A254 (144.6083, -13.7108) -> (146.1048, -13.8128) centre (145.3565, -13.7618) ccw
  line L256 (144.6083, -13.7108) -> (144.6477, -13.1322)
  arc A255 (146.1442, -13.2342) -> (144.6477, -13.1322) centre (145.396, -13.1832) ccw
  line L257 (121.4624, -33.6767) -> (120.6514, -35.1366)
  arc A256 (119.3402, -34.4083) -> (120.6514, -35.1366) centre (119.9958, -34.7725) ccw
  line L258 (119.3402, -34.4083) -> (120.1511, -32.9484)
  arc A257 (121.4624, -33.6767) -> (120.1511, -32.9484) centre (120.8067, -33.3125) ccw
  line L259 (127.0942, -32.2842) -> (127.0548, -32.8628)
  arc A258 (125.5583, -32.7608) -> (127.0548, -32.8628) centre (126.3065, -32.8118) ccw
  line L260 (125.5583, -32.7608) -> (125.5977, -32.1822)
  arc A259 (127.0942, -32.2842) -> (125.5977, -32.1822) centre (126.346, -32.2332) ccw
  line L261 (140.5123, 42.5233) -> (139.7014, 41.0634)
  arc A260 (138.3902, 41.7917) -> (139.7014, 41.0634) centre (139.0458, 41.4275) ccw
  line L262 (138.3902, 41.7917) -> (139.2011, 43.2516)
  arc A261 (140.5123, 42.5233) -> (139.2011, 43.2516) centre (139.8567, 42.8875) ccw
  line L263 (146.1442, 43.9158) -> (146.1048, 43.3372)
  arc A262 (144.6083, 43.4392) -> (146.1048, 43.3372) centre (145.3565, 43.3882) ccw
  line L264 (144.6083, 43.4392) -> (144.6477, 44.0178)
  arc A263 (146.1442, 43.9158) -> (144.6477, 44.0178) centre (145.396, 43.9668) ccw
  line L265 (140.5123, 23.4733) -> (139.7014, 22.0134)
  arc A264 (138.3902, 22.7417) -> (139.7014, 22.0134) centre (139.0458, 22.3775) ccw
  line L266 (138.3902, 22.7417) -> (139.2011, 24.2016)
  arc A265 (140.5123, 23.4733) -> (139.2011, 24.2016) centre (139.8567, 23.8375) ccw
  line L267 (146.1442, 24.8658) -> (146.1048, 24.2872)
  arc A266 (144.6083, 24.3892) -> (146.1048, 24.2872) centre (145.3565, 24.3382) ccw
  line L268 (144.6083, 24.3892) -> (144.6477, 24.9678)
  arc A267 (146.1442, 24.8658) -> (144.6477, 24.9678) centre (145.396, 24.9168) ccw
  line L269 (140.5123, -33.6767) -> (139.7014, -35.1366)
  arc A268 (138.3902, -34.4083) -> (139.7014, -35.1366) centre (139.0458, -34.7725) ccw
  line L270 (138.3902, -34.4083) -> (139.2011, -32.9484)
  arc A269 (140.5123, -33.6767) -> (139.2011, -32.9484) centre (139.8567, -33.3125) ccw
  line L271 (146.1442, -32.2842) -> (146.1048, -32.8628)
  arc A270 (144.6083, -32.7608) -> (146.1048, -32.8628) centre (145.3565, -32.8118) ccw
  line L272 (144.6083, -32.7608) -> (144.6477, -32.1822)
  arc A271 (146.1442, -32.2842) -> (144.6477, -32.1822) centre (145.396, -32.2332) ccw
  line L273 (102.4124, -33.6767) -> (101.6014, -35.1366)
  arc A272 (100.2902, -34.4083) -> (101.6014, -35.1366) centre (100.9458, -34.7725) ccw
  line L274 (100.2902, -34.4083) -> (101.1011, -32.9484)
  arc A273 (102.4124, -33.6767) -> (101.1011, -32.9484) centre (101.7567, -33.3125) ccw
  line L275 (108.0442, -32.2842) -> (108.0048, -32.8628)
  arc A274 (106.5083, -32.7608) -> (108.0048, -32.8628) centre (107.2565, -32.8118) ccw
  line L276 (106.5083, -32.7608) -> (106.5477, -32.1822)
  arc A275 (108.0442, -32.2842) -> (106.5477, -32.1822) centre (107.296, -32.2332) ccw
  line L277 (95.2686, -14.6267) -> (94.4577, -16.0866)
  arc A276 (93.1464, -15.3583) -> (94.4577, -16.0866) centre (93.802, -15.7225) ccw
  line L278 (93.1464, -15.3583) -> (93.9573, -13.8984)
  arc A277 (95.2686, -14.6267) -> (93.9573, -13.8984) centre (94.613, -14.2625) ccw
  line L279 (100.9005, -13.2342) -> (100.861, -13.8128)
  arc A278 (99.3645, -13.7108) -> (100.861, -13.8128) centre (100.1128, -13.7618) ccw
  line L280 (99.3645, -13.7108) -> (99.404, -13.1322)
  arc A279 (100.9005, -13.2342) -> (99.404, -13.1322) centre (100.1522, -13.1832) ccw
  circle A280 centre (-138.9938, 34.125) radius 0.35
  circle A281 centre (-146.7937, 34.125) radius 0.35
  circle A282 centre (-112.8, -42.075) radius 0.35
  circle A283 centre (-120.6, -42.075) radius 0.35
  circle A284 centre (-88.9875, -42.075) radius 0.35
  circle A285 centre (-96.7875, -42.075) radius 0.35
  circle A286 centre (-100.8938, 34.125) radius 0.35
  circle A287 centre (-108.6937, 34.125) radius 0.35
  circle A288 centre (-91.3688, 15.075) radius 0.35
  circle A289 centre (-99.1688, 15.075) radius 0.35
  circle A290 centre (-86.6063, -3.975) radius 0.35
  circle A291 centre (-94.4062, -3.975) radius 0.35
  circle A292 centre (-77.0812, -23.025) radius 0.35
  circle A293 centre (-84.8812, -23.025) radius 0.35
  circle A294 centre (-81.8438, 34.125) radius 0.35
  circle A295 centre (-89.6438, 34.125) radius 0.35
  circle A296 centre (-72.3187, 15.075) radius 0.35
  circle A297 centre (-80.1188, 15.075) radius 0.35
  circle A298 centre (-67.5563, -3.975) radius 0.35
  circle A299 centre (-75.3563, -3.975) radius 0.35
  circle A300 centre (-58.0313, -23.025) radius 0.35
  circle A301 centre (-65.8312, -23.025) radius 0.35
  circle A302 centre (-134.2312, 15.075) radius 0.35
  circle A303 centre (-142.0312, 15.075) radius 0.35
  circle A304 centre (-62.7938, 34.125) radius 0.35
  circle A305 centre (-70.5938, 34.125) radius 0.35
  circle A306 centre (-53.2688, 15.075) radius 0.35
  circle A307 centre (-61.0688, 15.075) radius 0.35
  circle A308 centre (-48.5063, -3.975) radius 0.35
  circle A309 centre (-56.3063, -3.975) radius 0.35
  circle A310 centre (-38.9813, -23.025) radius 0.35
  circle A311 centre (-46.7813, -23.025) radius 0.35
  circle A312 centre (-43.7437, 34.125) radius 0.35
  circle A313 centre (-51.5438, 34.125) radius 0.35
  circle A314 centre (-34.2188, 15.075) radius 0.35
  circle A315 centre (-42.0188, 15.075) radius 0.35
  circle A316 centre (-29.4563, -3.975) radius 0.35
  circle A317 centre (-37.2563, -3.975) radius 0.35
  circle A318 centre (-19.9312, -23.025) radius 0.35
  circle A319 centre (-27.7313, -23.025) radius 0.35
  circle A320 centre (-131.85, -3.975) radius 0.35
  circle A321 centre (-139.65, -3.975) radius 0.35
  circle A322 centre (-24.6938, 34.125) radius 0.35
  circle A323 centre (-32.4937, 34.125) radius 0.35
  circle A324 centre (-15.1687, 15.075) radius 0.35
  circle A325 centre (-22.9688, 15.075) radius 0.35
  circle A326 centre (-10.4063, -3.975) radius 0.35
  circle A327 centre (-18.2063, -3.975) radius 0.35
  circle A328 centre (-0.8813, -23.025) radius 0.35
  circle A329 centre (-8.6813, -23.025) radius 0.35
  circle A330 centre (-17.55, -42.075) radius 0.35
  circle A331 centre (-25.35, -42.075) radius 0.35
  circle A332 centre (-5.6437, 34.125) radius 0.35
  circle A333 centre (-13.4438, 34.125) radius 0.35
  circle A334 centre (3.8813, 15.075) radius 0.35
  circle A335 centre (-3.9188, 15.075) radius 0.35
  circle A336 centre (8.6438, -3.975) radius 0.35
  circle A337 centre (0.8438, -3.975) radius 0.35
  circle A338 centre (18.1687, -23.025) radius 0.35
  circle A339 centre (10.3688, -23.025) radius 0.35
  circle A340 centre (-127.0875, -23.025) radius 0.35
  circle A341 centre (-134.8875, -23.025) radius 0.35
  circle A342 centre (13.4063, 34.125) radius 0.35
  circle A343 centre (5.6063, 34.125) radius 0.35
  circle A344 centre (22.9312, 15.075) radius 0.35
  circle A345 centre (15.1313, 15.075) radius 0.35
  circle A346 centre (27.6938, -3.975) radius 0.35
  circle A347 centre (19.8938, -3.975) radius 0.35
  circle A348 centre (37.2188, -23.025) radius 0.35
  circle A349 centre (29.4187, -23.025) radius 0.35
  circle A350 centre (32.4562, 34.125) radius 0.35
  circle A351 centre (24.6562, 34.125) radius 0.35
  circle A352 centre (41.9813, 15.075) radius 0.35
  circle A353 centre (34.1812, 15.075) radius 0.35
  circle A354 centre (46.7438, -3.975) radius 0.35
  circle A355 centre (38.9438, -3.975) radius 0.35
  circle A356 centre (56.2687, -23.025) radius 0.35
  circle A357 centre (48.4688, -23.025) radius 0.35
  circle A358 centre (-136.6125, -42.075) radius 0.35
  circle A359 centre (-144.4125, -42.075) radius 0.35
  circle A360 centre (51.5063, 34.125) radius 0.35
  circle A361 centre (43.7062, 34.125) radius 0.35
  circle A362 centre (61.0312, 15.075) radius 0.35
  circle A363 centre (53.2313, 15.075) radius 0.35
  circle A364 centre (65.7938, -3.975) radius 0.35
  circle A365 centre (57.9938, -3.975) radius 0.35
  circle A366 centre (75.3187, -23.025) radius 0.35
  circle A367 centre (67.5187, -23.025) radius 0.35
  circle A368 centre (51.5063, -42.075) radius 0.35
  circle A369 centre (43.7062, -42.075) radius 0.35
  circle A370 centre (70.5563, 34.125) radius 0.35
  circle A371 centre (62.7563, 34.125) radius 0.35
  circle A372 centre (80.0812, 15.075) radius 0.35
  circle A373 centre (72.2812, 15.075) radius 0.35
  circle A374 centre (84.8438, -3.975) radius 0.35
  circle A375 centre (77.0438, -3.975) radius 0.35
  circle A376 centre (101.5125, -23.025) radius 0.35
  circle A377 centre (93.7125, -23.025) radius 0.35
  circle A378 centre (-119.9437, 34.125) radius 0.35
  circle A379 centre (-127.7438, 34.125) radius 0.35
  circle A380 centre (70.5563, -42.075) radius 0.35
  circle A381 centre (62.7563, -42.075) radius 0.35
  circle A382 centre (89.6063, 34.125) radius 0.35
  circle A383 centre (81.8063, 34.125) radius 0.35
  circle A384 centre (99.1313, 15.075) radius 0.35
  circle A385 centre (91.3312, 15.075) radius 0.35
  circle A386 centre (115.8, -3.975) radius 0.35
  circle A387 centre (108, -3.975) radius 0.35
  circle A388 centre (127.7063, -23.025) radius 0.35
  circle A389 centre (119.9063, -23.025) radius 0.35
  circle A390 centre (89.6063, -42.075) radius 0.35
  circle A391 centre (81.8063, -42.075) radius 0.35
  circle A392 centre (118.1813, 34.125) radius 0.35
  circle A393 centre (110.3813, 34.125) radius 0.35
  circle A394 centre (122.9438, 15.075) radius 0.35
  circle A395 centre (115.1438, 15.075) radius 0.35
  circle A396 centre (146.7562, -3.975) radius 0.35
  circle A397 centre (138.9563, -3.975) radius 0.35
  circle A398 centre (146.7562, -23.025) radius 0.35
  circle A399 centre (138.9563, -23.025) radius 0.35
  circle A400 centre (-110.4188, 15.075) radius 0.35
  circle A401 centre (-118.2188, 15.075) radius 0.35
  circle A402 centre (127.7063, -42.075) radius 0.35
  circle A403 centre (119.9063, -42.075) radius 0.35
  circle A404 centre (146.7562, 34.125) radius 0.35
  circle A405 centre (138.9563, 34.125) radius 0.35
  circle A406 centre (146.7562, 15.075) radius 0.35
  circle A407 centre (138.9563, 15.075) radius 0.35
  circle A408 centre (108.6563, -42.075) radius 0.35
  circle A409 centre (100.8563, -42.075) radius 0.35
  circle A410 centre (146.7562, -42.075) radius 0.35
  circle A411 centre (138.9563, -42.075) radius 0.35
  circle A412 centre (-105.6562, -3.975) radius 0.35
  circle A413 centre (-113.4562, -3.975) radius 0.35
  circle A414 centre (-96.1312, -23.025) radius 0.35
  circle A415 centre (-103.9313, -23.025) radius 0.35
  circle A416 centre (143, 52.5) radius 2.15
  circle A417 centre (143, -52) radius 2.15
  circle A418 centre (-144.75, 52.5) radius 2.15
  circle A419 centre (-140.5, -52.5) radius 2.15
  circle A420 centre (-142.8938, 38.8875) radius 1.994
  circle A421 centre (-147.9737, 38.8875) radius 0.851
  circle A422 centre (-137.8137, 38.8875) radius 0.851
  circle A423 centre (-116.7, -37.3125) radius 1.994
  circle A424 centre (-121.78, -37.3125) radius 0.851
  circle A425 centre (-111.62, -37.3125) radius 0.851
  circle A426 centre (-92.8875, -37.3125) radius 1.994
  circle A427 centre (-97.9675, -37.3125) radius 0.851
  circle A428 centre (-87.8075, -37.3125) radius 0.851
  circle A429 centre (-104.7938, 38.8875) radius 1.994
  circle A430 centre (-109.8738, 38.8875) radius 0.851
  circle A431 centre (-99.7138, 38.8875) radius 0.851
  circle A432 centre (-95.2688, 19.8375) radius 1.994
  circle A433 centre (-100.3487, 19.8375) radius 0.851
  circle A434 centre (-90.1887, 19.8375) radius 0.851
  circle A435 centre (-90.5062, 0.7875) radius 1.994
  circle A436 centre (-95.5863, 0.7875) radius 0.851
  circle A437 centre (-85.4262, 0.7875) radius 0.851
  circle A438 centre (-80.9813, -18.2625) radius 1.994
  circle A439 centre (-86.0613, -18.2625) radius 0.851
  circle A440 centre (-75.9013, -18.2625) radius 0.851
  circle A441 centre (-85.7438, 38.8875) radius 1.994
  circle A442 centre (-90.8238, 38.8875) radius 0.851
  circle A443 centre (-80.6637, 38.8875) radius 0.851
  circle A444 centre (-76.2188, 19.8375) radius 1.994
  circle A445 centre (-81.2987, 19.8375) radius 0.851
  circle A446 centre (-71.1388, 19.8375) radius 0.851
  circle A447 centre (-71.4562, 0.7875) radius 1.994
  circle A448 centre (-76.5362, 0.7875) radius 0.851
  circle A449 centre (-66.3762, 0.7875) radius 0.851
  circle A450 centre (-61.9313, -18.2625) radius 1.994
  circle A451 centre (-67.0113, -18.2625) radius 0.851
  circle A452 centre (-56.8513, -18.2625) radius 0.851
  circle A453 centre (-138.1312, 19.8375) radius 1.994
  circle A454 centre (-143.2113, 19.8375) radius 0.851
  circle A455 centre (-133.0513, 19.8375) radius 0.851
  circle A456 centre (-66.6937, 38.8875) radius 1.994
  circle A457 centre (-71.7738, 38.8875) radius 0.851
  circle A458 centre (-61.6138, 38.8875) radius 0.851
  circle A459 centre (-57.1688, 19.8375) radius 1.994
  circle A460 centre (-62.2488, 19.8375) radius 0.851
  circle A461 centre (-52.0887, 19.8375) radius 0.851
  circle A462 centre (-52.4063, 0.7875) radius 1.994
  circle A463 centre (-57.4863, 0.7875) radius 0.851
  circle A464 centre (-47.3263, 0.7875) radius 0.851
  circle A465 centre (-42.8813, -18.2625) radius 1.994
  circle A466 centre (-47.9612, -18.2625) radius 0.851
  circle A467 centre (-37.8013, -18.2625) radius 0.851
  circle A468 centre (-47.6438, 38.8875) radius 1.994
  circle A469 centre (-52.7238, 38.8875) radius 0.851
  circle A470 centre (-42.5637, 38.8875) radius 0.851
  circle A471 centre (-38.1187, 19.8375) radius 1.994
  circle A472 centre (-43.1987, 19.8375) radius 0.851
  circle A473 centre (-33.0388, 19.8375) radius 0.851
  circle A474 centre (-33.3563, 0.7875) radius 1.994
  circle A475 centre (-38.4363, 0.7875) radius 0.851
  circle A476 centre (-28.2763, 0.7875) radius 0.851
  circle A477 centre (-23.8313, -18.2625) radius 1.994
  circle A478 centre (-28.9113, -18.2625) radius 0.851
  circle A479 centre (-18.7512, -18.2625) radius 0.851
  circle A480 centre (-135.75, 0.7875) radius 1.994
  circle A481 centre (-140.83, 0.7875) radius 0.851
  circle A482 centre (-130.67, 0.7875) radius 0.851